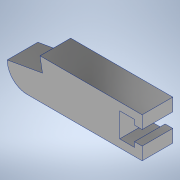
# Autodesk Inventor part: Finray_test_8_Kerbe_10deg
Saved by Autodesk Inventor 2022 (Build 260153000, 153)
## iProperties
Created: 2022-02-28
Part Number: Finray_test_8_Kerbe_10deg
Material: Generic
Document SubType Name: Modeling
Designer: richa
Density: 1 g/cm^3
Appearance: Aluminum - Flat
Author: richa
Autodesk Inventor part; units mm, degrees
ref_plane "YZ Plane" through (0, 0, 0) normal (1, 0, 0) x (0, 1, 0)
ref_plane "XZ Plane" through (0, 0, 0) normal (0, 1, 0) x (-1, 0, 0)
ref_plane "XY Plane" through (0, 0, 0) normal (0, 0, 1) x (1, 0, 0)
sketch "Sketch5" plane through (0, 0, 0) normal (0, 0, 1) x (1, 0, 0)
  line L0 (52.8, -15.6) -> (52.8, -10.6)
  line L1 (52.8, -10.6) -> (49.8, -10.6)
  line L2 (49.8, -10.6) -> (49.8, -12.55)
  line L3 (44, -12.55) -> (44, -3.05)
  line L4 (49.8, -3.05) -> (49.8, -5)
  line L5 (49.8, -5) -> (52.8, -5)
  line L6 (52.8, -5) -> (52.8, 0)
  line L7 (52.8, 0) -> (7.8, 0)
  line L8 (44, -3.05) -> (49.8, -3.05)
  line L9 (44, -12.55) -> (49.8, -12.55)
  line L10 (52.8, -15.6) -> (7.8, -15.6)
  arc A0 (7.8, 0) -> (7.8, -15.6) centre (7.8, -7.8) ccw
  point P0 (0, 0)
  dimension "d41" = 5.8
  dimension "d48" = 44
  dimension "d50" = 3
  dimension "d63" = 45
  dimension "d67" = 15.6
  dimension "d71" = 0
  dimension "d72" = 36.2
  dimension "d87" = 5.6
  dimension "d88" = 9.5
  constraints: 22 end point, 7 perpendicular, 4 collinear, 2 parallel, 2 point on circle, 2 tangent, 1 centre point, 1 horizontal, 1 vertical
  measures "d41" distance between parallel lines of L2 L3
  measures "d48" distance from line of L3 point (0, 0)
  measures "d50" distance of L4.end L5.end
  measures "d63" distance of L0.start L10.end
  measures "d67" diameter of A0
  measures "d71" distance from line of point (0, 0) L7
  measures "d72" distance from line of L3 A0.centre
  measures "d87" distance from line of L0.end L5
  measures "d88" distance of L3.start L3.end
extrude "Extrusion2" add sketch "Sketch5" along normal blind 12
sketch "Sketch8" plane through (0, 0, 0) normal (0, 0, -1) x (-1, 0, 0)
  arc A0 (-7.8, -15.6) -> (-7.8, 0) centre (-7.8, -7.8) ccw projected
  line L0 (-12.8406, 0) -> (-13.7873, -5.3689)
  line L1 (-7.8, 0) -> (-1.143, 0) construction
  arc A1 (-7.8, -15.6) -> (-7.8, 0) centre (-7.8, -7.8) ccw projected
  line L2 (-7.8, -7.8) -> (4.6142, -7.8) construction
  line L3 (1.4517, -9.4313) -> (-7.8, -7.8) construction
  line L4 (-7.8, -7.8) -> (-18.1105, -5.982) construction
  line L5 (-52.8, 0) -> (-7.8, 0) projected
  arc A2 (-0.1185, -9.1545) -> (-7.8, 0) centre (-7.8, -7.8) ccw
  line L6 (0, -7.8) -> (-13.7873, -5.3689)
  line L7 (-52.8, 0) -> (-7.8, 0) projected
  line L8 (-7.8, 0) -> (-12.8406, 0)
  point P0 (0, 0)
  point P1 (-9.1339, -7.5648)
  dimension "d80" = 100
  dimension "d81" = 10
  dimension "d89" = 14
  constraints: 14 end point, 4 point on circle, 4 point on line, 2 horizontal, 1 centre point, 1 concentric, 1 perpendicular
  measures "d80" angle of L0 L1
  measures "d81" angle of L2 L3
  measures "d89" distance of L6.start L0.end
extrude "Extrusion5" cut sketch "Sketch8" against normal through all
equation "\"l1\" = 8"
body "Solid2"
